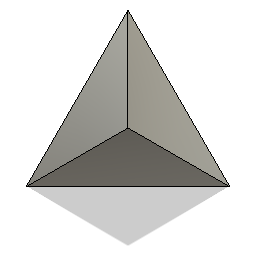
Tetrahedron_v1 (Autodesk Fusion 360 design; units mm, degrees)
Autodesk Fusion 360 part; units mm, degrees
sketch "Sketch1" plane through (0, 0, 0) normal (0, 1, 0) x (1, 0, 0)
  line L0 (50, 50) -> (-50, 50)
  line L1 (-50, 50) -> (-50, -50)
  line L2 (-50, -50) -> (50, -50)
  line L3 (50, -50) -> (50, 50)
  line L4 (50, 50) -> (-50, -50) construction
  line L5 (-50, 50) -> (50, -50) construction
  dimension "d1" = 100
extrude "Extrude1" add sketch "Sketch1" along normal mid plane 100
sketch "Sketch2" plane through (0, 0, -50) normal (0, 0, -1) x (-1, 0, 0)
  line L0 (50, -50) -> (50, 50)
  line L1 (50, 50) -> (-50, 50)
  line L2 (-50, 50) -> (-50, -50)
  line L3 (-50, -50) -> (50, -50)
  line L4 (-50, -50) -> (50, 50)
  line L5 (50, 50, 0) -> (-50, 50, -100)
  line L6 (-50, 50, -100) -> (-50, -50, 0)
  line L7 (-50, -50, 0) -> (50, -50, -100)
  line L8 (50, -50, -100) -> (-50, 50, -100)
  line L9 (50, -50, -100) -> (50, 50, 0)
ref_plane "WorkPlane1" through (50, 50, 50) normal (-0.57735, -0.57735, 0.57735) x (0.707107, -0.707107, 0)
sketch "Sketch3" plane through (50, 50, 50) normal (-0.57735, -0.57735, 0.57735) x (0.707107, -0.707107, 0)
  line L0 (-70.7107, -122.4745) -> (0, 0)
  line L1 (0, 0) -> (70.7107, -122.4745)
  line L2 (70.7107, -122.4745) -> (-70.7107, -122.4745)
extrude "Extrude2" cut sketch "Sketch3" against normal blind 80
ref_plane "WorkPlane2" through (-50, 50, -50) normal (0.57735, 0.57735, 0.57735) x (-0.707107, 0.707107, 0)
sketch "Sketch4" plane through (-50, 50, -50) normal (0.57735, 0.57735, 0.57735) x (-0.707107, 0.707107, 0)
  line L0 (-70.7107, 122.4745) -> (0, 0)
  line L1 (-141.4214, 0) -> (0, 0)
  line L2 (-141.4214, 0) -> (-70.7107, 122.4745)
extrude "Extrude3" cut sketch "Sketch2" along normal blind 150 contours L4 L7 L9 in plane through (0, 0, -50) normal (-0.57735, -0.57735, -0.57735)
ref_plane "WorkPlane3" through (50, 50, 50) normal (-0.57735, 0.57735, 0.57735) x (-0.707107, -0.707107, 0)
sketch "Sketch5" plane through (50, 50, 50) normal (-0.57735, 0.57735, 0.57735) x (-0.707107, -0.707107, 0)
  line L0 (70.7107, -122.4745) -> (0, 0)
  line L1 (141.4214, 0) -> (70.7107, -122.4745)
  line L2 (141.4214, 0) -> (0, 0)
extrude "Extrude4" cut sketch "Sketch2" along normal blind 150 contours L5 L8 L9 in plane through (-33.3333, 33.3333, -16.6667) normal (-0.57735, 0.57735, 0.57735)
ref_plane "WorkPlane4" through (50, 50, 50) normal (0.57735, -0.57735, 0.57735) x (0.707107, 0.707107, 0)
sketch "Sketch6" plane through (50, 50, 50) normal (0.57735, -0.57735, 0.57735) x (0.707107, 0.707107, 0)
  line L0 (-141.4214, 0) -> (0, 0)
  line L1 (0, 0) -> (-70.7107, -122.4745)
  line L2 (-70.7107, -122.4745) -> (-141.4214, 0)
extrude "Extrude5" cut sketch "Sketch6" along normal blind 105
